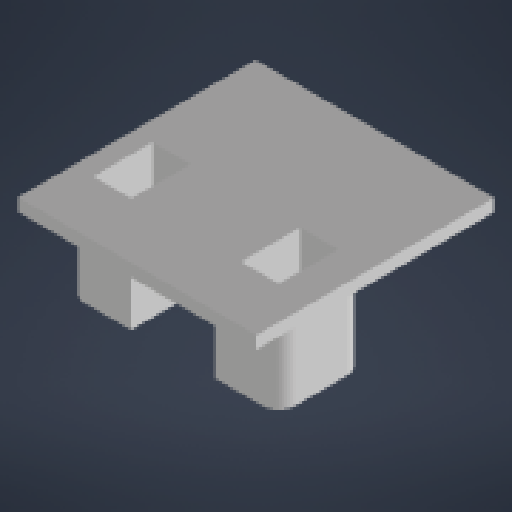
# Autodesk Inventor part: tail_box
Saved by Autodesk Inventor 2024 (Build 280153000, 153)
## iProperties
Created: 2023-05-16
Part Number: tail_box
Material: Типовые
Document SubType Name: Modeling
Designer: user
Density: 1 g/cm^3
Appearance: По умолчанию
Author: user
Autodesk Inventor part; units mm, degrees
ref_plane "YZ Plane" through (0, 0, 0) normal (1, 0, 0) x (0, 1, 0)
ref_plane "XZ Plane" through (0, 0, 0) normal (0, 1, 0) x (-1, 0, 0)
ref_plane "XY Plane" through (0, 0, 0) normal (0, 0, 1) x (1, 0, 0)
sketch "Эскиз1" plane through (0, 0, 0) normal (0, 0, 1) x (1, 0, 0)
  line L0 (0, 0) -> (15, 0)
  line L1 (15, 0) -> (15, 20)
  line L2 (15, 20) -> (0, 20)
  line L3 (0, 20) -> (0, 0)
  line L4 (35, 20) -> (50, 20)
  line L5 (50, 20) -> (50, 0)
  line L6 (50, 0) -> (35, 0)
  line L7 (35, 0) -> (35, 20)
  circle A0 centre (7.5, 10) radius 2
  circle A1 centre (42.5, 10) radius 2
  point P0 (7.5, 20)
  point P1 (15, 10)
  point P2 (35, 10)
  point P3 (42.5, 20)
  dimension "d0" = 4
  dimension "d1" = 15
  dimension "d2" = 20
  dimension "d3" = 20
  constraints: 16 end point, 4 midpoint, 4 parallel, 2 centre point, 2 equal length, 2 horizontal, 2 horizontal alignment, 2 perpendicular, 2 vertical alignment, 1 equal radius, 1 point on line
  measures "d0" diameter of A0
  measures "d1" distance of L1.end L2.end
  measures "d2" distance of L0.end L1.end
  measures "d3" distance of L4.start L1.end
extrude "Выдавливание1" add sketch "Эскиз1" along normal blind 4
sketch "Эскиз2" plane through (0, 0, 4) normal (0, 0, 1) x (1, 0, 0)
  line L0 (15, 0) -> (15, 20) projected
  line L1 (15, 20) -> (0, 20) projected
  line L2 (0, 20) -> (0, 0) projected
  line L3 (0, 0) -> (15, 0) projected
  line L4 (35, 0) -> (50, 0) projected
  line L5 (50, 0) -> (50, 20) projected
  line L6 (50, 20) -> (35, 20) projected
  line L7 (35, 20) -> (35, 0) projected
  line L8 (3, 17) -> (12, 17)
  line L9 (12, 17) -> (12, 3)
  line L10 (12, 3) -> (3, 3)
  line L11 (3, 3) -> (3, 17)
  line L12 (38, 17) -> (47, 17)
  line L13 (47, 17) -> (47, 3)
  line L14 (47, 3) -> (38, 3)
  line L15 (38, 3) -> (38, 17)
  dimension "d6" = 3
  dimension "d7" = 3
  constraints: 16 end point, 6 other
  measures "d6" distance between parallel lines of L1 L8
  measures "d7" distance between parallel lines of L6 L12
extrude "Выдавливание2" add sketch "Эскиз2" along normal blind 17
fillet "Сопряжение1" radius 4 4 edges at (0, 0, 10.5) (50, 0, 10.5) (50, 20, 10.5) (0, 20, 10.5)
sketch "Эскиз3" plane through (0, 0, 21) normal (0, 0, 1) x (1, 0, 0)
  line L0 (-7.5, 50) -> (57.5, 50)
  line L1 (57.5, 50) -> (57.5, -20)
  line L2 (57.5, -20) -> (-7.5, -20)
  line L3 (-7.5, -20) -> (-7.5, 50)
  line L4 (3, 17) -> (12, 17) projected
  line L5 (3, 3) -> (3, 17) projected
  line L6 (12, 3) -> (3, 3) projected
  line L7 (12, 17) -> (12, 3) projected
  line L8 (38, 3) -> (38, 17) projected
  line L9 (38, 17) -> (47, 17) projected
  line L10 (47, 17) -> (47, 3) projected
  line L11 (47, 3) -> (38, 3) projected
  line L12 (12, 10) -> (38, 10) construction
  point P0 (0, 0)
  point P1 (25, 10)
  point P2 (25, -20)
  point P3 (-7.5, 15)
  dimension "d15" = 65
  dimension "d16" = 70
  dimension "d17" = 30
  constraints: 10 end point, 5 midpoint, 2 parallel, 1 horizontal, 1 perpendicular, 1 vertical alignment
  measures "d15" distance of L1.end L2.end
  measures "d16" distance of L2.end L0.start
  measures "d17" vertical distance of L1.end point (25, 10)
extrude "Выдавливание3" add sketch "Эскиз3" along normal blind 3
sketch "Эскиз4" plane through (4, 20, 0) normal (0, 1, 0) x (1, 0, 0)
  circle A0 centre (4.5, -10) radius 4 projected
  circle A1 centre (37.5, -10) radius 4 projected
  point P0 (-4, 0)
extrude "Выдавливание4" cut sketch "Эскиз4" against normal through all
sketch "Эскиз5" plane through (0, 0, 24) normal (0, 0, 1) x (1, 0, 0)
  line L0 (-7.5, 50) -> (-7.5, -20) projected
  line L1 (-7.5, -20) -> (57.5, -20) projected
  line L2 (57.5, -20) -> (57.5, 50) projected
  line L3 (57.5, 50) -> (-7.5, 50) projected
  line L4 (-4.5, -17) -> (-4.5, 47)
  line L5 (-4.5, 47) -> (54.5, 47)
  line L6 (54.5, 47) -> (54.5, -17)
  line L7 (54.5, -17) -> (-4.5, -17)
  point P0 (0, 0)
  dimension "d18" = 3
  constraints: 8 end point, 3 other
  measures "d18" distance between parallel lines of L0 L4
extrude "Выдавливание5" add sketch "Эскиз5" along normal blind 77.5
sketch "Эскиз6" plane through (-7.5, -20, 21) normal (0, -1, 0) x (1, 0, 0)
  line L0 (3, 3) -> (62, 3) projected
  line L1 (3, 3) -> (3, 80.5) projected
  line L2 (62, 80.5) -> (3, 80.5) projected
  line L3 (62, 3) -> (62, 80.5) projected
  point P0 (7.5, -21)
extrude "Выдавливание6" cut sketch "Эскиз6" against normal blind 5
sketch "Эскиз7" plane through (54.5, -20, 24) normal (-1, 0, 0) x (0, 0, 1)
  line L0 (77.5, 0) -> (69.5, 0)
  line L1 (69.5, 0) -> (69.5, 8)
  line L2 (69.5, 8) -> (77.5, 8)
  line L3 (77.5, 8) -> (77.5, 0)
  line L4 (77.5, 0) -> (0, 0) projected
  circle A0 centre (73.5, 4) radius 1.95
  point P0 (-24, 20)
  point P1 (77.5, 4)
  point P2 (73.5, 8)
  dimension "d25" = 8
  dimension "d26" = 8
  dimension "d27" = 3.9
  constraints: 8 end point, 2 midpoint, 2 parallel, 1 centre point, 1 horizontal, 1 horizontal alignment, 1 perpendicular, 1 vertical alignment
  measures "d25" distance of L1.end L2.end
  measures "d26" distance of L0.end L1.end
  measures "d27" diameter of A0
extrude "Выдавливание7" add sketch "Эскиз7" along normal blind 3
sketch "Эскиз8" plane through (54.5, -16, 97.5) normal (-1, 0, 0) x (0, 0, 1)
  circle A0 centre (0, 0) radius 1.95 projected
  point P0 (-97.5, 16)
extrude "Выдавливание8" cut sketch "Эскиз8" against normal blind 5
ref_plane "РабПлоскость1" through (25, -20, 21) normal (-1, 0, 0) x (0, 0, 1)
mirror "Зеркальное отражение1" about plane through (25, -20, 21) normal (-1, 0, 0) of "Выдавливание7", "Выдавливание8"
fillet "Сопряжение3" radius 4 9 edges at (-7.5, 50, 61.25) (57.5, 50, 61.25) (-4.5, 47, 62.75) (54.5, 47, 62.75) (57.5, 15, 21) (-7.5, 15, 21) (-4.5, 13.5, 24) (25, 47, 24) (54.5, 13.5, 24)
fillet "Сопряжение4" radius 4 3 edges at (-6.3284, 48.8284, 22.1716) (56.3284, 48.8284, 22.1716) (25, 50, 21)
equation "\"d26\" = d25"
